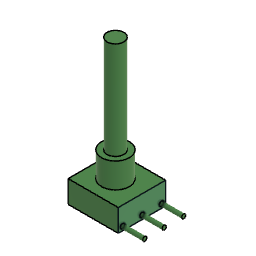
Potentiometer v3 (Autodesk Fusion 360 design; units mm, degrees)
Autodesk Fusion 360 part; units mm, degrees
sketch "base" plane through (0, 0, 0) normal (0, 0, 1) x (1, 0, 0)
  line L0 (0, 0) -> (18, 0)
  line L1 (18, 0) -> (18, 17)
  line L2 (18, 17) -> (0, 17)
  line L3 (0, 17) -> (0, 0)
  dimension "d1" = 17
  dimension "d2" = 18
  constraint horizontal L0
  constraint vertical L1
  constraint horizontal L2
  constraint vertical L3
  constraint coincident L0.start L3.end
  measures "d1" distance of L0.start L2.end
  measures "d2" distance of L0.start L0.end
extrude "Extrude1" add sketch "base" along normal blind 8
sketch "pins" plane through (18, 0, 0) normal (1, 0, 0) x (0, 1, 0)
  line L0 (0, 0) -> (17, 0)
  line L1 (17, 0) -> (17, 8)
  line L2 (17, 8) -> (0, 8)
  line L3 (0, 8) -> (0, 0)
  circle A0 centre (1.5, 1.5) radius 0.75
  circle A1 centre (8.5, 1.5) radius 0.75
  circle A2 centre (15.5, 1.5) radius 0.75
  dimension "d5" = 1.5
  dimension "d6" = 1.5
  dimension "d7" = 1.5
  dimension "d12" = 14
  dimension "d13" = 0
  measures "d5" diameter of A0
  measures "d6" distance of L0 A0.centre
  measures "d7" distance of L3 A0.centre
extrude "Extrude3" add sketch "pins" along normal blind 8 contours A0 | A1 | A2
sketch "base knob" plane through (0, 0, 8) normal (0, 0, 1) x (-1, 0, 0)
  line L0 (0, -17) -> (0, 0)
  line L1 (0, 0) -> (-18, 0)
  line L2 (-18, 0) -> (-18, -17)
  line L3 (-18, -17) -> (0, -17)
  circle A0 centre (-8.5, -8.5) radius 5
  dimension "d16" = 10
  dimension "d17" = 8.5
  dimension "d18" = 8.5
  measures "d16" diameter of A0
  measures "d17" distance of L3 A0.centre
  measures "d18" distance of L0 A0.centre
extrude "Extrude4" add sketch "base knob" along normal blind 9 contours A0
sketch "knob" plane through (0, 0, 17) normal (0, 0, 1) x (-1, 0, 0)
  circle A0 centre (-8.5, -8.5) radius 5
  circle A1 centre (-8.5, -8.5) radius 3
  dimension "d21" = 6
  constraint concentric A0 A1
  measures "d21" diameter of A1
extrude "Extrude5" add sketch "knob" along normal blind 35 contours A1
equation "d18 = d17"
